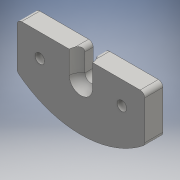
# Autodesk Inventor part: Kameralefogov3
Saved by Autodesk Inventor 2016 (Build 200138000, 138)
## iProperties
Created: 2018-03-31
Part Number: Kameralefogov3
Material: Generic
Document SubType Name: Modeling
Designer: bogna
Density: 1 g/cm^3
Appearance: Default
Author: bogna
Autodesk Inventor part; units mm, degrees
ref_plane "YZ Plane" through (0, 0, 0) normal (1, 0, 0) x (0, 1, 0)
ref_plane "XZ Plane" through (0, 0, 0) normal (0, 1, 0) x (-1, 0, 0)
ref_plane "XY Plane" through (0, 0, 0) normal (0, 0, 1) x (1, 0, 0)
sketch "Sketch1" plane through (0, 0, 0) normal (0, 1, 0) x (-1, 0, 0)
  line L0 (0, -28.84) -> (0, 33.04) projected
  line L1 (39.2, 0) -> (-39.2, 0) projected
  line L2 (-28, 10) -> (-28, -10)
  line L3 (28, 10) -> (28, -10)
  line L4 (-28, 10) -> (-2.6, 10)
  line L5 (-2.6, 10) -> (-2.6, 0)
  line L6 (28, 10) -> (2.6, 10)
  line L7 (2.6, 10) -> (2.6, 0)
  arc A0 (-2.6, 0) -> (2.6, 0) centre (0, 0) ccw
  arc A1 (-28, -10) -> (28, -10) centre (0, 24.2) ccw
  dimension "d0" = 5.2
  dimension "d1" = 56
  dimension "d2" = 20
  dimension "d3" = 10
  dimension "d4" = 20
  constraints: 12 end point, 4 point on circle, 2 centre point, 2 horizontal, 2 perpendicular, 2 vertical, 1 collinear, 1 parallel, 1 tangent, 2 other
  measures "d0" distance between parallel lines of L7 L5
  measures "d1" distance between parallel lines of L3 L2
  measures "d2" distance of L2.start L2.end
  measures "d3" distance of L4.end L5.end
  measures "d4" distance edge to line of A1 L1
extrude "Extrusion1" add sketch "Sketch1" along normal blind 8 contours A1 L2 L1 A0 L0 | L0 A0 L1 L3 A1 | L1 L2 L4 L5 | L7 L6 L3 L1
sketch "Sketch2" plane through (0, 0, 0) normal (0, 0, 1) x (1, 0, 0)
  arc A0 (5.1, 0) -> (0, 5.1) centre (0, 0) ccw
  line L0 (0, -1.2312) -> (0, 7.3875) projected
  line L1 (0, 5.1) -> (0, 0)
  line L2 (0, 0) -> (5.1, 0)
  dimension "d7" = 10.2
  constraints: 4 end point, 2 point on circle, 1 centre point, 1 coincident, 1 collinear, 1 perpendicular, 1 point on line
  measures "d7" diameter of A0
revolve "Revolution1" cut sketch "Sketch2" angle 360 about axis through (0, -10, 0) along (0, 1, 0)
sketch "Sketch4" plane through (0, 8, 0) normal (0, 1, 0) x (1, 0, 0)
  line L0 (0, 26) -> (0, -16) projected
  line L1 (28, -10) -> (28, 10) projected
  line L2 (39.2, 0) -> (-39.2, 0) projected
  point P0 (0, 0)
  point P1 (18, 0)
  point P2 (-18, 0)
  dimension "d9" = 10
  constraints: 1 point on line, 1 symmetric about line
  measures "d9" distance from line of L1 point (18, 0)
hole "Hole1" at (18, 8, 0) at (-18, 8, 0) direction (0, -1, 0) diameter 4.2 end through all counterbore diameter 8.65 counterbore depth 3.1
fillet "Fillet1" radius 2 6 edges at (28, 4, 10) (28, 4, -10) (-28, 4, -10) (-28, 4, 10) (-2.6, 4, 10) (2.6, 4, 10)
sketch "Sketch5" plane through (0, 0, 0) normal (0, 0, 1) x (1, 0, 0)
  line L0 (4.6, 0) -> (26, 0) projected
  arc A0 (5.1, 0) -> (-5.1, 0) centre (0, 0) ccw
  line L1 (5.1, 0) -> (-5.1, 0) projected
  line L2 (-5.1, 0) -> (5.1, 0)
  point P0 (2.6, 0)
  point P1 (-2.6, 0)
  dimension "d18" = 5.1
  constraints: 2 end point, 2 point on circle, 1 centre point, 1 coincident, 1 collinear, 1 point on line
  measures "d18" radius of A0
extrude "Extrusion2" cut sketch "Sketch5" along normal blind 10
body "Solid1"
